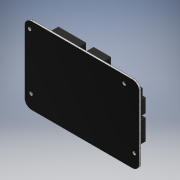
# Autodesk Inventor part: Teensy And Breakout
Saved by Autodesk Inventor 2018 (Build 220112000, 112)
## iProperties
Created: 2018-09-04
Part Number: Teensy And Breakout
Material: Generic
Document SubType Name: Modeling
Designer: matth
Density: 1 g/cm^3
Appearance: Default
Author: matth
Autodesk Inventor part; units mm, degrees
ref_plane "YZ Plane" through (0, 0, 0) normal (1, 0, 0) x (0, 1, 0)
ref_plane "XZ Plane" through (0, 0, 0) normal (0, 1, 0) x (-1, 0, 0)
ref_plane "XY Plane" through (0, 0, 0) normal (0, 0, 1) x (1, 0, 0)
sketch "Sketch1" plane through (0, 0, 0) normal (0, 1, 0) x (-1, 0, 0)
  line L0 (0, 0) -> (-4.3, 0)
  line L1 (-4.3, 0) -> (-4.3, -12)
  line L2 (-4.3, -12) -> (95.7, -12)
  line L3 (95.7, -12) -> (95.7, 55)
  line L4 (95.7, 55) -> (-4.3, 55)
  line L5 (-4.3, 55) -> (-4.3, 0)
  circle A0 centre (0, 0) radius 1.5
  line L6 (0, 0) -> (90.17, 0)
  circle A1 centre (90.17, 0) radius 1.5
  line L7 (-4.3, 55) -> (-4.3, 48.26)
  line L8 (-4.3, 48.26) -> (8.89, 48.26)
  line L9 (8.89, 48.26) -> (91.44, 48.26)
  circle A2 centre (8.89, 48.26) radius 1.5
  circle A3 centre (91.44, 48.26) radius 1.5
  dimension "d0" = 4.3
  dimension "d1" = 12
  dimension "d2" = 100
  dimension "d3" = 67
  dimension "d4" = 3
  dimension "d5" = 90.17
  dimension "d6" = 3
  dimension "d7" = 6.74
  dimension "d8" = 13.19
  dimension "d9" = 82.55
  dimension "d10" = 3
  dimension "d11" = 3
  constraints: 20 end point, 4 centre point, 4 coincident, 4 horizontal, 4 perpendicular, 1 point on line, 1 vertical
  measures "d0" distance of L0.start L0.end
  measures "d1" distance of L0.end L1.end
  measures "d2" distance of L1.end L2.end
  measures "d3" distance of L2.end L3.end
  measures "d4" diameter of A0
  measures "d5" distance of L6.start L6.end
  measures "d6" diameter of A1
  measures "d7" distance of L4.end L7.end
  measures "d8" distance of L7.end L8.end
  measures "d9" distance of L8.end L9.end
  measures "d10" diameter of A2
  measures "d11" diameter of A3
extrude "Extrusion1" add sketch "Sketch1" along normal blind 1.5
fillet "Fillet1" radius 6 4 edges at (-95.7, 0.75, 55) (-95.7, 0.75, -12) (4.3, 0.75, -12) (4.3, 0.75, 55)
sketch "Sketch3" plane through (0, 1.5, 0) normal (0, 1, 0) x (1, 0, 0)
  line L0 (-80.2385, -43.3473) -> (-35.2385, -43.3473)
  line L1 (-35.2385, -43.3473) -> (-35.2385, -23.3473)
  line L2 (-35.2385, -23.3473) -> (-80.2385, -23.3473)
  line L3 (-80.2385, -23.3473) -> (-80.2385, -43.3473)
  line L4 (-35.2385, -43.3473) -> (-80.2385, -43.3473)
  line L5 (-80.2385, -43.3473) -> (-80.2385, -39.3473)
  line L6 (-80.2385, -39.3473) -> (-35.2385, -39.3473)
  line L7 (-35.2385, -39.3473) -> (-35.2385, -43.3473)
  line L8 (-35.2385, -23.3473) -> (-80.2385, -23.3473)
  line L9 (-80.2385, -23.3473) -> (-80.2385, -27.3473)
  line L10 (-80.2385, -27.3473) -> (-35.2385, -27.3473)
  line L11 (-35.2385, -27.3473) -> (-35.2385, -23.3473)
  point P0 (0, 0)
  dimension "d15" = 45
  dimension "d16" = 20
  dimension "d17" = 4
  dimension "d18" = 4
  constraints: 24 end point, 6 parallel, 3 horizontal, 3 perpendicular, 2 point on line
  measures "d15" distance of L2.end L1.end
  measures "d16" distance of L1.end L0.end
  measures "d17" distance of L4.end L5.end
  measures "d18" distance of L9.end L8.end
extrude "Extrusion2" add sketch "Sketch3" along normal blind 8 contours L3 L6 L1 L0 | L3 L2 L1 L10
sketch "Sketch4" plane through (0, 9.5, 0) normal (0, 1, 0) x (1, 0, 0)
  line L0 (-80.2385, -39.3473) -> (-80.2385, -43.3473) projected
  line L1 (-80.2385, -43.3473) -> (-81.2385, -43.3473)
  line L2 (-81.2385, -43.3473) -> (-81.2385, -44.3473)
  line L3 (-81.2385, -44.3473) -> (-34.2385, -44.3473)
  line L4 (-34.2385, -44.3473) -> (-34.2385, -22.3473)
  line L5 (-34.2385, -22.3473) -> (-81.2385, -22.3473)
  line L6 (-81.2385, -22.3473) -> (-81.2385, -44.3473)
  point P0 (0, 0)
  dimension "d21" = 1
  dimension "d22" = 1
  dimension "d23" = 47
  dimension "d24" = 22
  constraints: 12 end point, 2 horizontal, 2 parallel, 2 perpendicular
  measures "d21" distance of L0.end L1.end
  measures "d22" distance of L1.end L2.end
  measures "d23" distance of L5.end L4.end
  measures "d24" distance of L4.end L3.end
extrude "Extrusion3" add sketch "Sketch4" along normal blind 1.5
sketch "Sketch5" plane through (0, 11, 0) normal (0, 1, 0) x (1, 0, 0)
  line L0 (-81.2385, -22.3473) -> (-81.2385, -44.3473) projected
  line L1 (-81.2385, -33.3473) -> (-76.2385, -33.3473)
  line L2 (-76.2385, -33.3473) -> (-76.2385, -31.3473)
  line L3 (-76.2385, -31.3473) -> (-81.2385, -31.3473)
  line L4 (-81.2385, -31.3473) -> (-81.2385, -33.3473)
  line L5 (-81.2385, -33.3473) -> (-76.2385, -33.3473)
  line L6 (-76.2385, -33.3473) -> (-76.2385, -35.3473)
  line L7 (-76.2385, -35.3473) -> (-81.2385, -35.3473)
  line L8 (-81.2385, -35.3473) -> (-81.2385, -33.3473)
  line L9 (-34.2385, -44.3473) -> (-34.2385, -22.3473) projected
  line L10 (-34.2385, -33.3473) -> (-36.2385, -33.3473)
  line L11 (-36.2385, -33.3473) -> (-36.2385, -29.3473)
  line L12 (-36.2385, -29.3473) -> (-34.2385, -29.3473)
  line L13 (-34.2385, -29.3473) -> (-34.2385, -33.3473)
  line L14 (-36.2385, -29.3473) -> (-44.2385, -29.3473)
  line L15 (-44.2385, -29.3473) -> (-44.2385, -37.3473)
  line L16 (-44.2385, -37.3473) -> (-36.2385, -37.3473)
  line L17 (-36.2385, -37.3473) -> (-36.2385, -29.3473)
  point P0 (0, 0)
  dimension "d27" = 5
  dimension "d28" = 2
  dimension "d29" = 2
  dimension "d30" = 2
  dimension "d31" = 4
  dimension "d32" = 8
  dimension "d33" = 8
  constraints: 32 end point, 8 parallel, 4 horizontal, 4 perpendicular, 2 midpoint
  measures "d27" distance of L3.end L2.end
  measures "d28" distance of L2.end L1.end
  measures "d29" distance of L5.end L6.end
  measures "d30" distance of L11.end L12.end
  measures "d31" distance of L10.end L11.end
  measures "d32" distance of L16.end L15.end
  measures "d33" distance of L15.end L14.end
extrude "Extrusion4" add sketch "Sketch5" along normal blind 3 contours L3 L2 L1 L0 | L1 L6 L7 L0 | L17 L16 L15 L14 L11
sketch "Sketch6" plane through (-81.2385, 9.5, 22.3473) normal (-1, 0, 0) x (0, 0, 1)
  line L0 (13, 1.5) -> (13, 4.5) projected
  line L1 (9, 1.5) -> (9, 4.5) projected
  line L2 (13, 4.5) -> (9, 4.5)
  line L3 (9, 4.5) -> (9, 1.5)
  line L4 (9, 1.5) -> (13, 1.5)
  line L5 (13, 1.5) -> (13, 4.5)
  point P0 (-22.3473, -9.5)
  constraints: 8 end point, 2 parallel, 1 horizontal, 1 perpendicular
extrude "Extrusion5" cut sketch "Sketch6" against normal blind 0.01
sketch "Sketch7" plane through (0, 1.5, 0) normal (0, 1, 0) x (1, 0, 0)
  line L0 (-89.7, -55) -> (-1.7, -55) projected
  line L1 (-75.8122, -55) -> (-73.8122, -55)
  line L2 (-75.8122, -55) -> (-75.8122, -53)
  line L3 (-75.8122, -53) -> (-51.8122, -53)
  line L4 (-51.8122, -53) -> (-51.8122, -47)
  line L5 (-51.8122, -47) -> (-75.8122, -47)
  line L6 (-75.8122, -47) -> (-75.8122, -53)
  line L7 (-45.0083, -55) -> (-45.0083, -53)
  line L8 (-45.0083, -53) -> (-30.0083, -53)
  line L9 (-30.0083, -53) -> (-30.0083, -47)
  line L10 (-30.0083, -47) -> (-45.0083, -47)
  line L11 (-45.0083, -47) -> (-45.0083, -53)
  line L12 (-23.232, -43.7266) -> (-11.232, -43.7266)
  line L13 (-11.232, -43.7266) -> (-11.232, -40.7266)
  line L14 (-11.232, -40.7266) -> (-23.232, -40.7266)
  line L15 (-23.232, -40.7266) -> (-23.232, -43.7266)
  line L16 (1.5411, -47.4426) -> (-3.4589, -47.4426)
  line L17 (-3.4589, -47.4426) -> (-3.4589, -40.4426)
  line L18 (-3.4589, -40.4426) -> (1.5411, -40.4426)
  line L19 (1.5411, -40.4426) -> (1.5411, -47.4426)
  line L20 (0.2226, -37.6132) -> (-2.7774, -37.6132)
  line L21 (-2.7774, -37.6132) -> (-2.7774, -25.6132)
  line L22 (-2.7774, -25.6132) -> (0.2226, -25.6132)
  line L23 (0.2226, -25.6132) -> (0.2226, -37.6132)
  line L24 (0.2226, -22.3296) -> (-2.7774, -22.3296)
  line L25 (-2.7774, -22.3296) -> (-2.7774, -4.3296)
  line L26 (-2.7774, -4.3296) -> (0.2226, -4.3296)
  line L27 (0.2226, -4.3296) -> (0.2226, -22.3296)
  line L28 (-7.2524, 7.9464) -> (-19.2524, 7.9464)
  line L29 (-19.2524, 7.9464) -> (-19.2524, 1.9464)
  line L30 (-19.2524, 1.9464) -> (-7.2524, 1.9464)
  line L31 (-7.2524, 1.9464) -> (-7.2524, 7.9464)
  line L32 (-24.7806, 7.9464) -> (-33.7806, 7.9464)
  line L33 (-33.7806, 7.9464) -> (-33.7806, 1.9464)
  line L34 (-33.7806, 1.9464) -> (-24.7806, 1.9464)
  line L35 (-24.7806, 1.9464) -> (-24.7806, 7.9464)
  line L36 (-42.8825, 7.9464) -> (-63.8825, 7.9464)
  line L37 (-63.8825, 7.9464) -> (-63.8825, 1.9464)
  line L38 (-63.8825, 1.9464) -> (-42.8825, 1.9464)
  line L39 (-42.8825, 1.9464) -> (-42.8825, 7.9464)
  line L40 (-68.9517, 7.9464) -> (-80.9517, 7.9464)
  line L41 (-80.9517, 7.9464) -> (-80.9517, 4.9464)
  line L42 (-80.9517, 4.9464) -> (-68.9517, 4.9464)
  line L43 (-68.9517, 4.9464) -> (-68.9517, 7.9464)
  line L44 (-89.7, -4.3296) -> (-86.7, -4.3296)
  line L45 (-86.7, -4.3296) -> (-86.7, -13.3296)
  line L46 (-86.7, -13.3296) -> (-89.7, -13.3296)
  line L47 (-89.7, -13.3296) -> (-89.7, -4.3296)
  line L48 (-76.8553, -9.2631) -> (-52.8553, -9.2631)
  line L49 (-52.8553, -9.2631) -> (-52.8553, -15.2631)
  line L50 (-52.8553, -15.2631) -> (-76.8553, -15.2631)
  line L51 (-76.8553, -15.2631) -> (-76.8553, -9.2631)
  point P0 (0, 0)
  dimension "d38" = 2
  dimension "d39" = 2
  dimension "d40" = 24
  dimension "d41" = 6
  dimension "d42" = 2
  dimension "d43" = 15
  dimension "d44" = 6
  dimension "d45" = 12
  dimension "d46" = 3
  dimension "d47" = 5
  dimension "d48" = 7
  dimension "d49" = 3
  dimension "d50" = 12
  dimension "d51" = 18
  dimension "d52" = 12
  dimension "d53" = 6
  dimension "d54" = 9
  dimension "d55" = 21
  dimension "d56" = 12
  dimension "d57" = 3
  dimension "d58" = 3
  dimension "d59" = 9
  dimension "d60" = 24
  dimension "d61" = 6
  constraints: 102 end point, 24 parallel, 12 horizontal, 12 perpendicular, 3 point on line, 2 vertical
  measures "d38" distance of L1.start L1.end
  measures "d39" distance of L1.start L2.end
  measures "d40" distance of L5.end L4.end
  measures "d41" distance of L4.end L3.end
  measures "d42" distance of L7.start L7.end
  measures "d43" distance of L10.end L9.end
  measures "d44" distance of L9.end L8.end
  measures "d45" distance of L14.end L13.end
  measures "d46" distance of L13.end L12.end
  measures "d47" distance of L17.end L18.end
  measures "d48" distance of L16.end L17.end
  measures "d49" distance of L21.end L22.end
  measures "d50" distance of L20.end L21.end
  measures "d51" distance of L24.end L25.end
  measures "d52" distance of L30.end L29.end
  measures "d53" distance of L29.end L28.end
  measures "d54" distance of L34.end L33.end
  measures "d55" distance of L38.end L37.end
  measures "d56" distance of L42.end L41.end
  measures "d57" distance of L41.end L40.end
  measures "d58" distance of L45.end L46.end
  measures "d59" distance of L44.end L45.end
  measures "d60" distance of L49.end L50.end
  measures "d61" distance of L48.end L49.end
extrude "Extrusion6" add sketch "Sketch7" along normal blind 8 contours L6 L5 L4 L3 | L11 L10 L9 L8 | L15 L14 L13 L12 | L20 L21 L22 L23 | L24 L25 L26 L27 | L31 L30 L29 L28 | L35 L34 L33 L32 | L39 L38 L37 L36 | L43 L42 L41 L40 | L44 L45 L46 L47 | L48 L49 L50 L51
extrude "Extrusion7" add sketch "Sketch7" along normal blind 4 contours L16 L17 L18 L19
body "Solid1"
